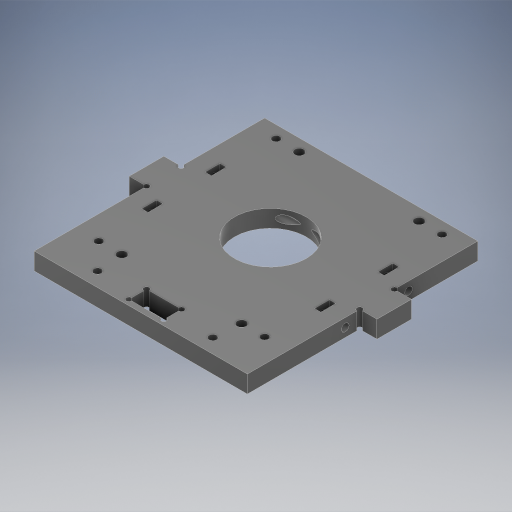
# Autodesk Inventor part: under the head
Saved by Autodesk Inventor 2024 (Build 280153000, 153)
## iProperties
Created: 2024-09-04
Part Number: under the head
Material: PMMA 플라스틱
Document SubType Name: Modeling
Designer: msi
Density: 1.188 g/cm^3
Appearance: 매끄러움 - 검은색
Mass: 40.9509 g
Surface Area: 159.801 cm^2
Volume: 34.4704 cm^3
Author: msi
Autodesk Inventor part; units mm, degrees
ref_plane "우측면도" through (0, 0, 0) normal (1, 0, 0) x (0, 1, 0)
ref_plane "평면도" through (0, 0, 0) normal (0, 1, 0) x (-1, 0, 0)
ref_plane "정면도" through (0, 0, 0) normal (0, 0, 1) x (1, 0, 0)
sketch "스케치1" plane through (0, 0, 0) normal (0, 1, 0) x (-1, 0, 0)
  line L0 (-37, 35) -> (37, 35)
  line L1 (37, 35) -> (37, -35)
  line L2 (37, -35) -> (-37, -35)
  line L3 (-37, -35) -> (-37, 35)
  line L4 (-37, 35) -> (37, -35) construction
  line L5 (37, 35) -> (-37, -35) construction
  line L6 (37, -14) -> (37, -2)
  line L7 (-37, -14) -> (-37, -2)
  line L8 (28.9, 13.6) -> (31.1, 13.6)
  line L9 (31.1, 13.6) -> (31.1, 8.4)
  line L10 (31.1, 8.4) -> (28.9, 8.4)
  line L11 (28.9, 8.4) -> (28.9, 13.6)
  line L12 (28.9, 13.6) -> (31.1, 8.4) construction
  line L13 (31.1, 13.6) -> (28.9, 8.4) construction
  line L14 (-31.1, 13.6) -> (-28.9, 13.6)
  line L15 (-28.9, 13.6) -> (-28.9, 8.4)
  line L16 (-28.9, 8.4) -> (-31.1, 8.4)
  line L17 (-31.1, 8.4) -> (-31.1, 13.6)
  line L18 (-31.1, 13.6) -> (-28.9, 8.4) construction
  line L19 (-28.9, 13.6) -> (-31.1, 8.4) construction
  line L20 (-31.1, -8.4) -> (-28.9, -8.4)
  line L21 (-28.9, -8.4) -> (-28.9, -13.6)
  line L22 (-28.9, -13.6) -> (-31.1, -13.6)
  line L23 (-31.1, -13.6) -> (-31.1, -8.4)
  line L24 (-31.1, -8.4) -> (-28.9, -13.6) construction
  line L25 (-28.9, -8.4) -> (-31.1, -13.6) construction
  line L26 (31.1, -8.4) -> (28.9, -8.4)
  line L27 (28.9, -8.4) -> (28.9, -13.6)
  line L28 (28.9, -13.6) -> (31.1, -13.6)
  line L29 (31.1, -13.6) -> (31.1, -8.4)
  line L30 (31.1, -8.4) -> (28.9, -13.6) construction
  line L31 (28.9, -8.4) -> (31.1, -13.6) construction
  line L32 (37, 6) -> (43, 6)
  line L33 (43, 6) -> (43, -6)
  line L34 (43, -6) -> (37, -6)
  line L35 (37, -6) -> (37, 6)
  line L36 (-37, 6) -> (-43, 6)
  line L37 (-43, 6) -> (-43, -6)
  line L38 (-43, -6) -> (-37, -6)
  line L39 (-37, -6) -> (-37, 6)
  circle A0 centre (20.8, 30.8) radius 1.6
  circle A1 centre (20.8, -30.8) radius 1.6
  circle A2 centre (-20.8, 30.8) radius 1.6
  circle A3 centre (-20.8, -30.8) radius 1.6
  circle A4 centre (28.8, 30.8) radius 1.35
  circle A5 centre (28.8, -30.8) radius 1.35
  circle A6 centre (-28.8, 30.8) radius 1.35
  circle A7 centre (-28.8, -30.8) radius 1.35
  point P0 (0, 0)
  point P1 (30, 11)
  point P2 (-30, 11)
  point P3 (-30, -11)
  point P4 (30, -11)
  dimension "d0" = 74
  dimension "d1" = 70
  dimension "d6" = 2.2
  dimension "d7" = 5.2
  dimension "d8" = 2.2
  dimension "d9" = 5.2
  dimension "d10" = 2.2
  dimension "d11" = 5.2
  dimension "d12" = 2.2
  dimension "d13" = 5.2
  dimension "d14" = 6
  dimension "d15" = 12
  dimension "d16" = 6
  dimension "d17" = 12
  dimension "d18" = 3.2
  dimension "d19" = 4.2
  dimension "d20" = 3.2
  dimension "d21" = 3.2
  dimension "d22" = 3.2
  dimension "d23" = 2.7
  dimension "d24" = 2.7
  dimension "d25" = 2.7
  dimension "d26" = 2.7
  constraints: 80 end point, 14 parallel, 10 midpoint, 8 centre point, 7 horizontal, 7 perpendicular, 4 point on line
  measures "d0" distance of L1.end L2.end
  measures "d1" distance of L0.end L1.end
  measures "d6" distance of L9.end L10.end
  measures "d7" distance of L8.end L9.end
  measures "d8" distance of L15.end L16.end
  measures "d9" distance of L14.end L15.end
  measures "d10" distance of L21.end L22.end
  measures "d11" distance of L20.end L21.end
  measures "d12" distance of L28.end L27.end
  measures "d13" distance of L27.end L26.end
  measures "d14" distance of L33.end L34.end
  measures "d15" distance of L32.end L33.end
  measures "d16" distance of L38.end L37.end
  measures "d17" distance of L37.end L36.end
  measures "d18" diameter of A0
  measures "d19" distance from line of L0 A0.centre
  measures "d20" diameter of A1
  measures "d21" diameter of A2
  measures "d22" diameter of A3
  measures "d23" diameter of A4
  measures "d24" diameter of A5
  measures "d25" diameter of A6
  measures "d26" diameter of A7
extrude "돌출1" add sketch "스케치1" along normal blind 6
sketch "스케치2" plane through (37, 0, 35) normal (1, 0, 0) x (0, 0, -1)
  circle A0 centre (46, 3) radius 1.35
  circle A1 centre (24, 3) radius 1.35
  point P0 (35, 0)
  dimension "d29" = 2.7
  dimension "d30" = 2.7
  constraints: 2 centre point
  measures "d29" diameter of A0
  measures "d30" diameter of A1
extrude "돌출2" cut sketch "스케치2" against normal blind 100
sketch "스케치3" plane through (-37, 0, 35) normal (0, 0, 1) x (1, 0, 0)
  line L0 (0, 0) -> (74, 0)
  line L1 (74, 0) -> (74, 6)
  line L2 (74, 6) -> (0, 6)
  line L3 (0, 6) -> (0, 0)
  point P0 (37, 0)
  dimension "d33" = 74
  dimension "d34" = 6
  constraints: 8 end point, 2 parallel, 1 horizontal, 1 perpendicular
  measures "d33" distance of L2.end L1.end
  measures "d34" distance of L1.end L0.end
extrude "돌출3" add sketch "스케치3" along normal blind 10
sketch "스케치4" plane through (0, 6, 0) normal (0, 1, 0) x (1, 0, 0)
  circle A0 centre (20, -40) radius 1.35
  circle A1 centre (-20, -40) radius 1.35
  line L0 (-6.05, -43.05) -> (6.05, -43.05)
  line L1 (6.05, -43.05) -> (6.05, -36.95)
  line L2 (6.05, -36.95) -> (-6.05, -36.95)
  line L3 (-6.05, -36.95) -> (-6.05, -43.05)
  line L4 (-6.05, -43.05) -> (6.05, -36.95) construction
  line L5 (6.05, -43.05) -> (-6.05, -36.95) construction
  point P0 (0, 0)
  point P1 (0, -40)
  dimension "d37" = 2.7
  dimension "d38" = 2.7
  dimension "d39" = 12.1
  dimension "d40" = 6.1
  constraints: 12 end point, 2 centre point, 2 midpoint, 2 parallel, 1 horizontal, 1 perpendicular
  measures "d37" diameter of A0
  measures "d38" diameter of A1
  measures "d39" distance of L2.end L1.end
  measures "d40" distance of L1.end L0.end
extrude "돌출4" cut sketch "스케치4" against normal blind 10
sketch "스케치5" plane through (0, 6, 0) normal (0, 1, 0) x (1, 0, 0)
  circle A0 centre (0, 0) radius 12.5
  dimension "d43" = 25
  constraints: 1 centre point, 1 coincident
  measures "d43" diameter of A0
extrude "돌출5" cut sketch "스케치5" against normal blind 10
sketch "스케치6" plane through (0, 6, 0) normal (0, 1, 0) x (1, 0, 0)
  circle A0 centre (0, 0) radius 12.5 projected
  circle A1 centre (20, -40) radius 1.35 projected
  circle A2 centre (-20, -40) radius 1.35 projected
  line L0 (-6.05, -36.95) -> (6.05, -36.95) projected
  line L1 (6.05, -36.95) -> (6.05, -43.05) projected
  line L2 (6.05, -43.05) -> (-6.05, -43.05) projected
  line L3 (-6.05, -43.05) -> (-6.05, -36.95) projected
  line L4 (37, -6) -> (37, -45) projected
  line L5 (37, -6) -> (43, -6) projected
  line L6 (43, -6) -> (43, 6) projected
  line L7 (43, 6) -> (37, 6) projected
  line L8 (37, 6) -> (37, 35) projected
  line L9 (37, 35) -> (-37, 35) projected
  line L10 (-37, 35) -> (-37, 6) projected
  line L11 (-37, 6) -> (-43, 6) projected
  line L12 (-43, 6) -> (-43, -6) projected
  line L13 (-43, -6) -> (-37, -6) projected
  line L14 (-37, -6) -> (-37, -45) projected
  line L15 (37, -45) -> (-37, -45) projected
  circle A3 centre (28.8, 30.8) radius 1.35 projected
  circle A4 centre (-28.8, 30.8) radius 1.35 projected
  circle A5 centre (-28.8, -30.8) radius 1.35 projected
  circle A6 centre (20.8, 30.8) radius 1.6 projected
  circle A7 centre (20.8, -30.8) radius 1.6 projected
  circle A8 centre (-20.8, 30.8) radius 1.6 projected
  circle A9 centre (-20.8, -30.8) radius 1.6 projected
  circle A10 centre (28.8, -30.8) radius 1.35 projected
  line L16 (-31.1, 8.4) -> (-31.1, 13.6) projected
  line L17 (-31.1, 13.6) -> (-28.9, 13.6) projected
  line L18 (-28.9, 13.6) -> (-28.9, 8.4) projected
  line L19 (-28.9, 8.4) -> (-31.1, 8.4) projected
  line L20 (31.1, 8.4) -> (28.9, 8.4) projected
  line L21 (28.9, 8.4) -> (28.9, 13.6) projected
  line L22 (28.9, 13.6) -> (31.1, 13.6) projected
  line L23 (31.1, 13.6) -> (31.1, 8.4) projected
  line L24 (31.1, -13.6) -> (28.9, -13.6) projected
  line L25 (28.9, -13.6) -> (28.9, -8.4) projected
  line L26 (28.9, -8.4) -> (31.1, -8.4) projected
  line L27 (31.1, -8.4) -> (31.1, -13.6) projected
  line L28 (-28.9, -13.6) -> (-31.1, -13.6) projected
  line L29 (-31.1, -13.6) -> (-31.1, -8.4) projected
  line L30 (-31.1, -8.4) -> (-28.9, -8.4) projected
  line L31 (-28.9, -8.4) -> (-28.9, -13.6) projected
  circle A11 centre (-6.05, -36.95) radius 1
  circle A12 centre (-6.05, -43.05) radius 1
  circle A13 centre (6.05, -36.95) radius 1
  circle A14 centre (6.05, -43.05) radius 1
  circle A15 centre (-37, -6) radius 1
  circle A16 centre (-37, 6) radius 1
  circle A17 centre (37, -6) radius 1
  circle A18 centre (37, 6) radius 1
  point P0 (38, -6)
  point P1 (37, -7)
  point P2 (37, 7)
  point P3 (38, 6)
  point P4 (-37, 7)
  point P5 (-38, 6)
  point P6 (-37, -7)
  point P7 (-38, -6)
  dimension "d46" = 2
  dimension "d47" = 2
  dimension "d48" = 2
  dimension "d49" = 2
  dimension "d50" = 2
  dimension "d51" = 2
  dimension "d52" = 2
  dimension "d53" = 2
  constraints: 8 centre point, 8 coincident
  measures "d46" diameter of A11
  measures "d47" diameter of A12
  measures "d48" diameter of A13
  measures "d49" diameter of A14
  measures "d50" diameter of A15
  measures "d51" diameter of A16
  measures "d52" diameter of A17
  measures "d53" diameter of A18
extrude "돌출6" cut sketch "스케치6" against normal through all contours L3 A11 L0 | L0 A11 L3 | A13 L1 L0 | L0 L1 A13 | A12 L2 L3 | L3 L2 A12 | A14 L2 L1 | L1 L2 A14 | L4 A17 L5 | L14 L13 A15 | A18 L8 L7 | L11 L10 A16 picked at (36.9727, -5.339) picked at (-37.657, -5.9202) picked at (36.9727, 5.339) picked at (-36.343, 5.9202)
